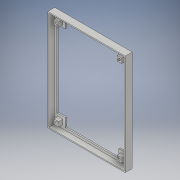
# Autodesk Inventor part: TestTapa_v0
Saved by Autodesk Inventor 2019 (Build 230136000, 136)
## iProperties
Created: 2019-05-27
Part Number: TestTapa_v0
Material: Genérico
Document SubType Name: Modeling
Designer: LuisAlonso
Density: 1 g/cm^3
Appearance: Valor por defecto
Author: LuisAlonso
Autodesk Inventor part; units mm, degrees
ref_plane "YZ Plane" through (0, 0, 0) normal (1, 0, 0) x (0, 1, 0)
ref_plane "XZ Plane" through (0, 0, 0) normal (0, 1, 0) x (-1, 0, 0)
ref_plane "XY Plane" through (0, 0, 0) normal (0, 0, 1) x (1, 0, 0)
sketch "Boceto1" plane through (0, 0, 0) normal (0, 0, 1) x (1, 0, 0)
  line L0 (-83, -108.2) -> (83, -108.2)
  line L1 (83, -108.2) -> (83, 108.2)
  line L2 (83, 108.2) -> (-83, 108.2)
  line L3 (-83, 108.2) -> (-83, -108.2)
  line L4 (-83, -108.2) -> (83, 108.2) construction
  line L5 (83, -108.2) -> (-83, 108.2) construction
  point P0 (0, 0)
  dimension "d0" = 166
  dimension "d1" = 216.4
  constraints: 12 end point, 2 midpoint, 2 parallel, 1 horizontal, 1 perpendicular
  measures "d0" distance of L2.end L1.end
  measures "d1" distance of L1.end L0.end
extrude "Extrusión1" add sketch "Boceto1" along normal blind 15
sketch "Boceto2" plane through (0, 0, 15) normal (0, 0, 1) x (1, 0, 0)
  line L0 (80.75, -105.95) -> (-80.75, -105.95)
  line L1 (-80.75, -105.95) -> (-80.75, 105.95)
  line L2 (80.75, 105.95) -> (-80.75, 105.95)
  line L3 (80.75, 105.95) -> (80.75, -105.95)
  line L4 (-83, 108.2) -> (83, 108.2)
  line L5 (83, 108.2) -> (83, -108.2)
  line L6 (83, -108.2) -> (-83, -108.2)
  line L7 (-83, -108.2) -> (-83, 108.2)
  point P0 (0, 0)
  constraints: 16 end point, 4 perpendicular, 2 parallel, 1 horizontal
extrude "Extrusión2" cut sketch "Boceto2" against normal blind 12 contours L0 L1 L2 L3
sketch "Boceto3" plane through (0, 0, 3) normal (0, 0, 1) x (1, 0, 0)
  line L0 (-67.5, -92.5) -> (67.5, -92.5)
  line L1 (67.5, -92.5) -> (67.5, 92.5)
  line L2 (67.5, 92.5) -> (-67.5, 92.5)
  line L3 (-67.5, 92.5) -> (-67.5, -92.5)
  line L4 (-62.5, 87.5) -> (-72.5, 87.5)
  line L5 (-72.5, 87.5) -> (-72.5, 97.5)
  line L6 (-72.5, 97.5) -> (-62.5, 97.5)
  line L7 (-62.5, 97.5) -> (-62.5, 87.5)
  line L8 (-62.5, 87.5) -> (-72.5, 97.5) construction
  line L9 (-72.5, 87.5) -> (-62.5, 97.5) construction
  line L10 (72.5, 87.5) -> (62.5, 87.5)
  line L11 (62.5, 87.5) -> (62.5, 97.5)
  line L12 (62.5, 97.5) -> (72.5, 97.5)
  line L13 (72.5, 97.5) -> (72.5, 87.5)
  line L14 (72.5, 87.5) -> (62.5, 97.5) construction
  line L15 (62.5, 87.5) -> (72.5, 97.5) construction
  line L16 (72.5, -97.5) -> (62.5, -97.5)
  line L17 (62.5, -97.5) -> (62.5, -87.5)
  line L18 (62.5, -87.5) -> (72.5, -87.5)
  line L19 (72.5, -87.5) -> (72.5, -97.5)
  line L20 (72.5, -97.5) -> (62.5, -87.5) construction
  line L21 (62.5, -97.5) -> (72.5, -87.5) construction
  line L22 (-62.5, -97.5) -> (-72.5, -97.5)
  line L23 (-72.5, -97.5) -> (-72.5, -87.5)
  line L24 (-72.5, -87.5) -> (-62.5, -87.5)
  line L25 (-62.5, -87.5) -> (-62.5, -97.5)
  line L26 (-62.5, -97.5) -> (-72.5, -87.5) construction
  line L27 (-72.5, -97.5) -> (-62.5, -87.5) construction
  point P0 (0, 0)
  dimension "d12" = 135
  dimension "d13" = 185
  dimension "d14" = 10
  dimension "d15" = 10
  dimension "d16" = 10
  dimension "d17" = 10
  dimension "d18" = 10
  dimension "d19" = 10
  dimension "d20" = 10
  dimension "d21" = 10
  constraints: 56 end point, 8 midpoint, 8 parallel, 6 perpendicular, 4 horizontal, 1 vertical
  measures "d12" distance of L0.start L0.end
  measures "d13" distance of L0.end L1.end
  measures "d14" distance of L5.end L6.end
  measures "d15" distance of L4.end L5.end
  measures "d16" distance of L11.end L12.end
  measures "d17" distance of L10.end L11.end
  measures "d18" distance of L17.end L18.end
  measures "d19" distance of L16.end L17.end
  measures "d20" distance of L23.end L24.end
  measures "d21" distance of L22.end L23.end
extrude "Extrusión3" add sketch "Boceto3" along normal blind 9 contours L3 L24 L25 L0 | L0 L25 L22 L23 L24 L3 | L17 L18 L1 L0 | L0 L1 L18 L19 L16 L17 | L4 L5 L6 L7 L2 L3 | L3 L2 L7 L4 | L10 L11 L2 L1 | L1 L2 L11 L12 L13 L10
sketch "Boceto4" plane through (0, 0, 0) normal (0, 0, -1) x (-1, 0, 0)
  line L0 (72.5, -97.5) -> (72.5, -87.5) projected
  line L1 (72.5, -87.5) -> (62.5, -87.5) projected
  line L2 (62.5, -87.5) -> (62.5, -97.5) projected
  line L3 (62.5, -97.5) -> (72.5, -97.5) projected
  line L4 (-62.5, 87.5) -> (-62.5, 97.5) projected
  line L5 (-62.5, 97.5) -> (-72.5, 97.5) projected
  line L6 (-72.5, 97.5) -> (-72.5, 87.5) projected
  line L7 (-72.5, 87.5) -> (-62.5, 87.5) projected
  line L8 (72.5, 87.5) -> (72.5, 97.5) projected
  line L9 (72.5, 97.5) -> (62.5, 97.5) projected
  line L10 (62.5, 97.5) -> (62.5, 87.5) projected
  line L11 (62.5, 87.5) -> (72.5, 87.5) projected
  line L12 (-62.5, -97.5) -> (-62.5, -87.5) projected
  line L13 (-62.5, -87.5) -> (-72.5, -87.5) projected
  line L14 (-72.5, -87.5) -> (-72.5, -97.5) projected
  line L15 (-72.5, -97.5) -> (-62.5, -97.5) projected
  line L16 (80.75, -105.95) -> (80.75, 105.95) projected
  line L17 (-80.75, -105.95) -> (80.75, -105.95) projected
  line L18 (-80.75, 105.95) -> (-80.75, -105.95) projected
  line L19 (80.75, 105.95) -> (-80.75, 105.95) projected
  line L20 (-67.5, -92.5) -> (-67.5, 92.5) projected
  line L21 (67.5, 92.5) -> (67.5, -92.5) projected
  line L22 (-67.5, 92.5) -> (67.5, 92.5) projected
  line L23 (67.5, -92.5) -> (-67.5, -92.5) projected
  circle A0 centre (-67.5, 92.5) radius 4.75
  circle A1 centre (67.5, 92.5) radius 4.75
  circle A2 centre (67.5, -92.5) radius 4.75
  circle A3 centre (-67.5, -92.5) radius 4.75
  point P0 (0, 0)
  dimension "d24" = 9.5
  dimension "d25" = 9.5
  dimension "d26" = 9.5
  dimension "d27" = 9.5
  constraints: 4 centre point, 4 coincident
  measures "d24" diameter of A0
  measures "d25" diameter of A1
  measures "d26" diameter of A2
  measures "d27" diameter of A3
extrude "Extrusión4" cut sketch "Boceto4" against normal blind 5.5 contours A2 L23 L21 | L21 L23 A2 | A1 L22 L21 | L21 L22 A1 | A3 L20 L23 | L23 L20 A3 | A0 L20 L22 | L22 L20 A0
sketch "Boceto5" plane through (67.5, 92.5, 5.5) normal (0, 0, -1) x (-1, 0, 0)
  arc A0 (2.2886, -0.8744) -> (0.8744, -2.2886) centre (0, 0) ccw
  line L0 (0, 0) -> (4.75, 0) construction
  line L1 (1.6679, -3.0821) -> (2.5764, -3.9906)
  line L2 (1.6679, -3.0821) -> (0.8744, -2.2886)
  line L3 (2.2886, -0.8744) -> (3.9906, -2.5764)
  arc A1 (2.5764, -3.9906) -> (3.9906, -2.5764) centre (0, 0) ccw
  line L4 (135, -185) -> (0, -185)
  arc A2 (134.1256, -2.2886) -> (132.7114, -0.8744) centre (135, 0) ccw
  line L5 (131.9179, -1.6679) -> (131.0094, -2.5764)
  line L6 (131.9179, -1.6679) -> (132.7114, -0.8744)
  line L7 (134.1256, -2.2886) -> (132.4236, -3.9906)
  arc A3 (131.0094, -2.5764) -> (132.4236, -3.9906) centre (135, 0) ccw
  arc A4 (132.7114, -184.1256) -> (134.1256, -182.7114) centre (135, -185) ccw
  line L8 (133.3321, -181.9179) -> (132.4236, -181.0094)
  line L9 (133.3321, -181.9179) -> (134.1256, -182.7114)
  line L10 (132.7114, -184.1256) -> (131.0094, -182.4236)
  arc A5 (132.4236, -181.0094) -> (131.0094, -182.4236) centre (135, -185) ccw
  arc A6 (0.8744, -182.7114) -> (2.2886, -184.1256) centre (0, -185) ccw
  line L11 (3.0821, -183.3321) -> (3.9906, -182.4236)
  line L12 (3.0821, -183.3321) -> (2.2886, -184.1256)
  line L13 (0.8744, -182.7114) -> (2.5764, -181.0094)
  arc A7 (3.9906, -182.4236) -> (2.5764, -181.0094) centre (0, -185) ccw
  point P0 (67.5, -92.5)
  dimension "d30" = 4.9
  dimension "d36" = 4.9
  dimension "d37" = 4.9
  dimension "d38" = 4.9
  constraints: 28 end point, 16 point on circle, 8 centre point, 1 horizontal
  measures "d30" diameter of A0
  measures "d36" diameter of A2
  measures "d37" diameter of A4
  measures "d38" diameter of A6
extrude "Extrusión5" cut sketch "Boceto5" against normal blind 10
sketch "Boceto6" plane through (0, 0, 3) normal (0, 0, 1) x (1, 0, 0)
  line L0 (62.5, -87.5) -> (62.5, -97.5) projected
  line L1 (72.5, -87.5) -> (62.5, -87.5) projected
  line L2 (-62.5, -97.5) -> (-62.5, -87.5) projected
  line L3 (-57.5, -97.5) -> (-57.5, -100.837)
  line L4 (-57.5, -100.837) -> (57.5, -100.837)
  line L5 (57.5, -100.837) -> (57.5, -82.5)
  line L6 (75.7581, -82.5) -> (57.5, -82.5)
  line L7 (-57.5, -100.837) -> (-57.5, -82.5)
  line L8 (-80.75, -105.95) -> (-80.75, 105.95) projected
  line L9 (75.7581, 82.5) -> (57.5081, 82.4907)
  line L10 (-80.75, 105.95) -> (80.75, 105.95) projected
  line L11 (57.5081, 105.95) -> (57.5081, 105.95)
  line L12 (57.5, -105.837) -> (57.5, -105.95)
  arc A0 (57.5, -105.837) -> (62.5, -100.837) centre (57.5, -100.837) ccw
  line L13 (62.5, -100.837) -> (62.5, -87.5)
  line L14 (72.5, -82.5) -> (75.7581, -82.5)
  line L15 (62.5, -87.5) -> (75.75, -87.5)
  line L16 (75.7581, -82.5) -> (75.7581, 82.5)
  arc A1 (75.8451, -87.4992) -> (80.7581, -82.5) centre (75.7581, -82.5) ccw
  arc A2 (80.7581, 82.5082) -> (75.75, 87.5) centre (75.7581, 82.5) ccw
  line L17 (62.5, 87.5) -> (72.5, 87.5) projected
  line L18 (75.75, 87.5) -> (62.5, 87.5)
  line L19 (62.5, 87.5) -> (62.5, 101.2352)
  line L20 (62.5, 97.5) -> (62.5, 87.5) projected
  arc A3 (62.5, 101.2352) -> (57.5081, 105.95) centre (57.5081, 100.95) ccw
  line L21 (57.5081, 82.4907) -> (57.5081, 100.95)
  line L22 (57.5081, 105.95) -> (57.5081, 105.95)
  arc A4 (-57.5, 105.95) -> (-62.5, 100.95) centre (-57.5, 100.95) ccw
  line L23 (-62.5, 87.5) -> (-62.5, 97.5) projected
  line L24 (-62.5, 100.95) -> (-62.5, 87.5)
  line L25 (-72.5, 97.5) -> (-72.5, 87.5) projected
  line L26 (-57.5, 82.5) -> (-57.5, 100.95)
  line L27 (-75.75, 82.5) -> (-75.75, -82.5)
  arc A5 (-75.75, 87.5) -> (-80.75, 82.5) centre (-75.75, 82.5) ccw
  line L28 (-75.75, 82.5) -> (-57.5, 82.5)
  line L29 (-62.5, 87.5) -> (-75.75, 87.5)
  line L30 (-62.5, -87.5) -> (-72.5, -87.5) projected
  arc A6 (-80.75, -82.5) -> (-75.75, -87.5) centre (-75.75, -82.5) ccw
  arc A7 (-62.5, -100.837) -> (-57.5, -105.837) centre (-57.5, -100.837) ccw
  line L31 (-75.75, -87.5) -> (-62.5, -87.5)
  line L32 (-62.5, -100.837) -> (-62.5, -87.5)
  line L33 (57.5, -105.837) -> (-57.5, -105.837)
  line L34 (80.75, -105.95) -> (-80.75, -105.95) projected
  line L35 (-80.75, -82.5) -> (-80.75, 82.5)
  line L36 (-57.5, 105.95) -> (57.5081, 105.95)
  line L37 (80.7581, 82.5082) -> (80.7581, -82.5)
  line L38 (-75.75, -82.5) -> (-57.5, -82.5)
  line L39 (57.5081, 100.95) -> (-57.5, 100.95)
  point P0 (0, 0)
  dimension "d52" = 5
  constraints: 58 end point, 17 point on circle, 8 centre point, 8 point on line, 6 collinear, 6 perpendicular, 6 vertical, 4 coincident, 4 horizontal, 2 parallel, 2 tangent
  measures "d52" distance of L27.start L35.end
extrude "Extrusión6" cut sketch "Boceto6" against normal blind 10 contours L7 L38 L27 L28 L26 L39 L21 L9 L16 L6 L5 L4 L3
